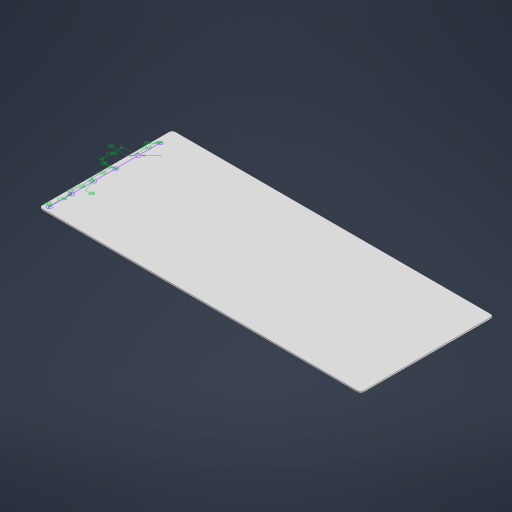
# Autodesk Inventor part: belly pan
Saved by Autodesk Inventor 2023 (Build 270158000, 158)
## iProperties
Created: 2023-11-20
Part Number: belly pan
Material: Generic
Document SubType Name: Modeling
Designer: Robodox
Density: 1 g/cm^3
Appearance: Default
Author: Robodox
Autodesk Inventor part; units mm, degrees
ref_plane "YZ Plane" through (0, 0, 0) normal (1, 0, 0) x (0, 1, 0)
ref_plane "XZ Plane" through (0, 0, 0) normal (0, 1, 0) x (-1, 0, 0)
ref_plane "XY Plane" through (0, 0, 0) normal (0, 0, 1) x (1, 0, 0)
sketch "Sketch1" plane through (0, 0, 0) normal (0, 1, 0) x (-1, 0, 0)
  line L0 (184.15, 76.2) -> (-184.15, 76.2)
  line L1 (-184.15, 76.2) -> (-184.15, -76.2)
  line L2 (-184.15, -76.2) -> (184.15, -76.2)
  line L3 (184.15, -76.2) -> (184.15, 76.2)
  point P0 (0, 0)
  point P1 (0, 0)
  dimension "d0" = 152.4
  dimension "d1" = 368.3
  constraints: 8 end point, 2 parallel, 1 coincident, 1 horizontal, 1 perpendicular
  measures "d0" distance of L2.end L0.start
  measures "d1" distance of L1.end L2.end
extrude "Extrusion1" add sketch "Sketch1" along normal blind 1.5875
fillet "Fillet1" radius 3.175 4 edges at (184.15, 0.7937, 76.2) (184.15, 0.7937, -76.2) (-184.15, 0.7937, 76.2) (-184.15, 0.7937, -76.2)
sketch "Sketch2" plane through (0, 1.5875, 0) normal (0, 1, 0) x (1, 0, 0)
  circle A0 centre (-178.5414, -70.5189) radius 2.54
  line L0 (-178.5414, -70.5189) -> (-178.5414, -45.1189)
  circle A1 centre (-178.5414, -45.1189) radius 2.54
  line L1 (-178.5414, -45.1189) -> (-178.5414, -19.7189)
  circle A2 centre (-178.5414, -19.7189) radius 2.54
  line L2 (-178.5414, -19.7189) -> (-178.5414, 5.6811)
  circle A3 centre (-178.5414, 5.6811) radius 2.54
  line L3 (-178.5414, 5.6811) -> (-178.5414, 31.0811)
  circle A4 centre (-178.5414, 31.0811) radius 2.54
  line L4 (-178.5414, 31.0811) -> (-178.5414, 56.4811)
  circle A5 centre (-178.5414, 56.4811) radius 2.54
  point P0 (0, 0)
  dimension "d7" = 5.08
  dimension "d8" = 25.4
  dimension "d9" = 5.08
  dimension "d10" = 25.4
  dimension "d11" = 5.08
  dimension "d12" = 25.4
  dimension "d13" = 5.08
  dimension "d14" = 25.4
  dimension "d15" = 5.08
  dimension "d16" = 25.4
  dimension "d17" = 5.08
  constraints: 10 end point, 6 centre point, 5 coincident, 4 vertical, 1 point on line
  measures "d7" diameter of A0
  measures "d8" distance of L0.start L0.end
  measures "d9" diameter of A1
  measures "d10" distance of L1.start L1.end
  measures "d11" diameter of A2
  measures "d12" distance of L2.start L2.end
  measures "d13" diameter of A3
  measures "d14" distance of L3.start L3.end
  measures "d15" diameter of A4
  measures "d16" distance of L4.start L4.end
  measures "d17" diameter of A5
body "Solid1"
